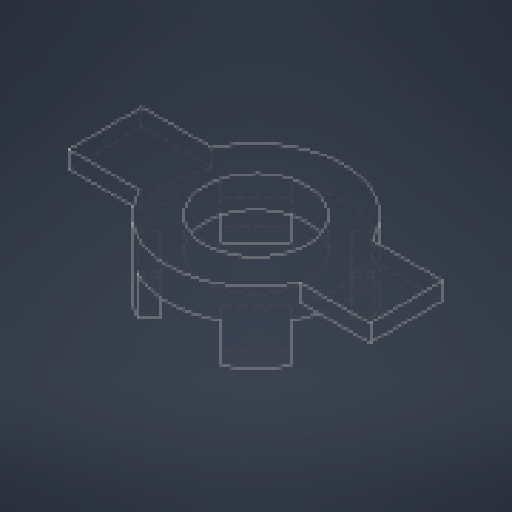
# Autodesk Inventor part: SistemLiberacion1
Saved by Autodesk Inventor 2026.1 (Build 301233000, 233)
## iProperties
Created: 2025-11-10
Part Number: SistemLiberacion1
Material: Genérico
Document SubType Name: Modeling
Designer: vickh
Density: 1 g/cm^3
Appearance: Valor por defecto
Author: vickh
Autodesk Inventor part; units mm, degrees
ref_plane "YZ Plane" through (0, 0, 0) normal (1, 0, 0) x (0, 1, 0)
ref_plane "XZ Plane" through (0, 0, 0) normal (0, 1, 0) x (-1, 0, 0)
ref_plane "XY Plane" through (0, 0, 0) normal (0, 0, 1) x (1, 0, 0)
sketch "Boceto1" plane through (0, 0, 0) normal (0, 1, 0) x (-1, 0, 0)
  circle A0 centre (0, 0) radius 10.5
  circle A1 centre (0, 0) radius 18
  dimension "d0" = 21
  dimension "d13" = 7.5
  constraints: 2 centre point, 2 coincident
  measures "d0" diameter of A0
  measures "d13" radial gap between concentric circles of A1 A0
extrude "Extrusión1" add sketch "Boceto1" along normal blind 11
sketch "Boceto2" plane through (0, 11, 0) normal (0, 1, 0) x (1, 0, 0)
  circle A0 centre (0, 0) radius 18 projected
  line L0 (-30.8631, -7.5) -> (-16.3631, -7.5)
  line L1 (-16.3631, 7.5) -> (-30.8631, 7.5)
  line L2 (-30.8631, 7.5) -> (-30.8631, -7.5)
  line L3 (-30.8631, -7.5) -> (-16.3631, 7.5) construction
  line L4 (-16.3631, -7.5) -> (-30.8631, 7.5) construction
  line L5 (30.8631, 7.5) -> (16.3631, 7.5)
  line L6 (16.3631, -7.5) -> (30.8631, -7.5)
  line L7 (30.8631, -7.5) -> (30.8631, 7.5)
  line L8 (30.8631, 7.5) -> (16.3631, -7.5) construction
  line L9 (16.3631, 7.5) -> (30.8631, -7.5) construction
  point P0 (-23.6131, 0)
  point P1 (23.6131, 0)
  point P2 (16.3631, 7.5)
  point P3 (16.3631, -7.5)
  dimension "d4" = 15
  dimension "d6" = 14.5
  dimension "d9" = 360
  dimension "d14" = 14.5
  constraints: 20 end point, 4 midpoint, 2 point on circle, 1 horizontal, 1 parallel, 1 vertical, 21 other
  measures "d4" distance of L0.end L1.start
  measures "d6" distance of L0.start L0.end
  measures "d14" distance of L1.start L1.end
extrude "Extrusión2" add sketch "Boceto2" along normal blind 3.5
sketch "Boceto3" plane through (0, 14.5, 0) normal (0, 1, 0) x (1, 0, 0)
  circle A0 centre (0, 0) radius 10.5
  dimension "d15" = 21
  constraints: 1 centre point, 1 coincident
  measures "d15" diameter of A0
extrude "Extrusión3" cut sketch "Boceto3" against normal blind 5
sketch "Boceto4" plane through (0, 0, 0) normal (0, -1, 0) x (1, 0, 0)
  circle A0 centre (0, 0) radius 18 projected
  line L0 (16.617, -9.5459) -> (9.5459, -16.617)
  line L1 (9.5459, -16.617) -> (6.1872, -13.2583)
  line L2 (6.1872, -13.2583) -> (13.2583, -6.1872)
  line L3 (13.2583, -6.1872) -> (16.617, -9.5459)
  line L4 (30.8631, 7.5) -> (30.8631, -7.5) construction
  line L5 (30.8631, 0) -> (-18, 0) construction
  line L6 (0, 25.0721) -> (0, -25.0721) construction
  line L7 (28.2843, -28.2843) -> (-28.2843, 28.2843) construction
  line L8 (35.3553, 35.3553) -> (-35.3553, -35.3553) construction
  line L9 (16.617, -9.5459) -> (6.1872, -13.2583) construction
  line L10 (13.2583, -6.1872) -> (9.5459, -16.617) construction
  line L11 (19.9536, -6.8721) -> (10.0541, 3.0274)
  circle A1 centre (0, 0) radius 10.5 projected
  line L12 (19.9536, -6.8721) -> (33.9536, -6.8721) construction
  line L13 (10.0541, 3.0274) -> (-3.0274, -10.0541)
  line L14 (-3.0274, -10.0541) -> (6.8721, -19.9536)
  line L15 (6.8721, -19.9536) -> (19.9536, -6.8721)
  line L16 (16.617, 9.5459) -> (13.2583, 6.1872)
  line L17 (9.5459, 16.617) -> (13.2583, 6.1872) construction
  line L18 (6.1872, 13.2583) -> (9.5459, 16.617)
  line L19 (6.1872, 13.2583) -> (16.617, 9.5459) construction
  line L20 (13.2583, 6.1872) -> (6.1872, 13.2583)
  line L21 (6.8721, 19.9536) -> (-3.0274, 10.0541)
  line L22 (10.0541, -3.0274) -> (19.9536, 6.8721)
  line L23 (9.5459, 16.617) -> (16.617, 9.5459)
  line L24 (19.9536, 6.8721) -> (6.8721, 19.9536)
  line L25 (-3.0274, 10.0541) -> (10.0541, -3.0274)
  line L26 (-9.5459, 16.617) -> (-6.1872, 13.2583)
  line L27 (-16.617, 9.5459) -> (-6.1872, 13.2583) construction
  line L28 (-13.2583, 6.1872) -> (-16.617, 9.5459)
  line L29 (-13.2583, 6.1872) -> (-9.5459, 16.617) construction
  line L30 (-6.1872, 13.2583) -> (-13.2583, 6.1872)
  line L31 (-19.9536, 6.8721) -> (-10.0541, -3.0274)
  line L32 (3.0274, 10.0541) -> (-6.8721, 19.9536)
  line L33 (-16.617, 9.5459) -> (-9.5459, 16.617)
  line L34 (-6.8721, 19.9536) -> (-19.9536, 6.8721)
  line L35 (-10.0541, -3.0274) -> (3.0274, 10.0541)
  line L36 (-16.617, -9.5459) -> (-13.2583, -6.1872)
  line L37 (-9.5459, -16.617) -> (-13.2583, -6.1872) construction
  line L38 (-6.1872, -13.2583) -> (-9.5459, -16.617)
  line L39 (-6.1872, -13.2583) -> (-16.617, -9.5459) construction
  line L40 (-13.2583, -6.1872) -> (-6.1872, -13.2583)
  line L41 (-6.8721, -19.9536) -> (3.0274, -10.0541)
  line L42 (-10.0541, 3.0274) -> (-19.9536, -6.8721)
  line L43 (-9.5459, -16.617) -> (-16.617, -9.5459)
  line L44 (-19.9536, -6.8721) -> (-6.8721, -19.9536)
  line L45 (3.0274, -10.0541) -> (-10.0541, 3.0274)
  point P0 (9.7227, -9.7227)
  point P1 (13.0815, -13.0815)
  point P2 (11.4021, -11.4021)
  point P3 (11.4021, 11.4021)
  point P4 (9.7227, 9.7227)
  point P5 (13.0815, 13.0815)
  point P6 (-11.4021, 11.4021)
  point P7 (-9.7227, 9.7227)
  point P8 (-13.0815, 13.0815)
  point P9 (-11.4021, -11.4021)
  point P10 (-9.7227, -9.7227)
  point P11 (-13.0815, -13.0815)
  point P12 (-15.7626, 8.6915)
  point P13 (-17.4595, 4.378)
  point P14 (-13.0815, 0)
  point P15 (-10.0541, 3.0274)
  point P16 (-3.0274, 10.0541)
  point P17 (0, 13.0815)
  point P18 (-4.378, 17.4595)
  point P19 (-8.6915, 15.7626)
  point P20 (15.7626, -8.6915)
  point P21 (17.4595, -4.378)
  point P22 (13.0815, 0)
  point P23 (10.0541, -3.0274)
  point P24 (3.0274, -10.0541)
  point P25 (0, -13.0815)
  point P26 (4.378, -17.4595)
  point P27 (8.6915, -15.7626)
  point P28 (8.6915, 15.7626)
  point P29 (4.378, 17.4595)
  point P30 (3.0274, 10.0541)
  point P31 (17.4595, 4.378)
  point P32 (15.7626, 8.6915)
  point P33 (-8.6915, -15.7626)
  point P34 (-4.378, -17.4595)
  point P35 (-10.0541, -3.0274)
  point P36 (-17.4595, -4.378)
  point P37 (-15.7626, -8.6915)
  dimension "d18" = 4.75
  dimension "d19" = 10
  dimension "d20" = 45
  dimension "d21" = 18.5
  dimension "d23" = 80
  dimension "d24" = 45
  dimension "d25" = 100
  dimension "d27" = 45
  dimension "d32" = 135
  dimension "d33" = 18.5
  dimension "d34" = 14
  dimension "d37" = 360
  constraints: 90 end point, 8 perpendicular, 7 midpoint, 2 point on circle, 1 coincident, 1 equal length, 1 horizontal, 1 point on line, 1 vertical, 87 other
  measures "d18" distance of point (9.723, -9.723) point (13.081, -13.081)
  measures "d19" distance of L1.end L2.end
  measures "d20" angle of L6 L2
  measures "d21" distance of point (0, 0) point (13.081, -13.081)
  measures "d23" distance of L7.start L7.end
  measures "d24" angle of L7 L6
  measures "d25" distance of L8.start L8.end
  measures "d27" angle of L8 L5
  measures "d32" angle of L12 L11
  measures "d33" distance between parallel lines of L14 L11
  measures "d34" distance between parallel lines of L13 L15
extrude "Extrusión4" cut sketch "Boceto4" against normal blind 8 contours A0 L11 L22 | L22 L11 A1 L32 L21 A0 L18 L20 L16 | A0 L3 L2 L1 L14 L41 A1 L22 L11 | L22 A1 L11 | L21 L32 A0 | A1 L21 L32 | L41 L14 A1 | A0 L41 L14 | L32 L21 A1 L42 L31 A0 L28 L30 L26 | L14 L41 A0 L38 L40 L36 L42 L31 A1 | A1 L31 L42 | L42 A0 L31
equation "\"d14\" = d6"
